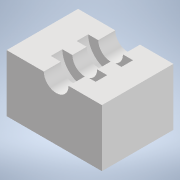
# Autodesk Inventor part: new_box_bottom
Saved by Autodesk Inventor 2021 (Build 250183000, 183)
## iProperties
Created: 2021-02-09
Part Number: new_box_bottom
Material: Generic
Document SubType Name: Modeling
Designer: user
Density: 1 g/cm^3
Appearance: Default
Author: user
Autodesk Inventor part; units mm, degrees
ref_plane "YZ Plane" through (0, 0, 0) normal (1, 0, 0) x (0, 1, 0)
ref_plane "XZ Plane" through (0, 0, 0) normal (0, 1, 0) x (-1, 0, 0)
ref_plane "XY Plane" through (0, 0, 0) normal (0, 0, 1) x (1, 0, 0)
sketch "Sketch1" plane through (0, 0, 0) normal (0, 1, 0) x (-1, 0, 0)
  line L0 (52, 58.6471) -> (-48, 58.6471)
  line L1 (-48, 58.6471) -> (-48, -16.3529)
  line L2 (-48, -16.3529) -> (52, -16.3529)
  line L3 (52, -16.3529) -> (52, 58.6471)
  point P0 (0, 0)
  dimension "d0" = 100
  dimension "d1" = 75
  constraints: 8 end point, 2 parallel, 1 horizontal, 1 perpendicular
  measures "d0" distance of L0.end L0.start
  measures "d1" distance of L1.end L0.end
extrude "Extrusion1" add sketch "Sketch1" along normal blind 60
sketch "Sketch2" plane through (0, 60, 0) normal (0, 1, 0) x (1, 0, 0)
  line L0 (-47, -53.6471) -> (43, -53.6471)
  line L1 (43, -53.6471) -> (43, 11.3529)
  line L2 (43, 11.3529) -> (-47, 11.3529)
  line L3 (-47, 11.3529) -> (-47, -53.6471)
  line L4 (-52, 16.3529) -> (-52, -58.6471) projected
  line L5 (-52, -58.6471) -> (48, -58.6471) projected
  line L6 (48, 16.3529) -> (-52, 16.3529) projected
  line L7 (48, -58.6471) -> (48, 16.3529) projected
  point P0 (0, 0)
  dimension "d4" = 5
  dimension "d5" = 5
  dimension "d6" = 5
  dimension "d7" = 5
  constraints: 8 end point, 2 parallel, 1 horizontal, 1 perpendicular
  measures "d4" distance from line of L4 L0.start
  measures "d5" distance between parallel lines of L5 L0
  measures "d6" distance between parallel lines of L6 L2
  measures "d7" distance between parallel lines of L7 L1
extrude "Extrusion2" cut sketch "Sketch2" against normal blind 59 contours L3 L2 L1 L0
sketch "Sketch3" plane through (48, 0, -16.3529) normal (0, 0, -1) x (-1, 0, 0)
  circle A0 centre (48, 60) radius 13
  point P0 (48, 0)
  dimension "d10" = 26
  dimension "d11" = 60
  constraints: 1 centre point
  measures "d10" diameter of A0
  measures "d11" distance of point (48, 0) A0.centre
sketch "Sketch13" plane through (0, 1, 0) normal (0, 1, 0) x (1, 0, 0)
  line L0 (-47, -53.6471) -> (-47, 11.3529) projected
  line L1 (43, 11.3529) -> (43, -53.6471) projected
  line L2 (-47, 11.3529) -> (43, 11.3529)
  line L3 (43, 11.3529) -> (43, -13.6471)
  line L4 (43, -13.6471) -> (-47, -13.6471)
  line L5 (-47, -13.6471) -> (-47, 11.3529)
  point P0 (0, 0)
  dimension "d44" = 25
  constraints: 8 end point, 2 parallel, 1 horizontal, 1 perpendicular, 1 point on line
  measures "d44" distance between parallel lines of L2 L4
extrude "Extrusion14" add sketch "Sketch13" along normal blind 59
sketch "Sketch14" plane through (-47, 1, 13.6471) normal (0, 0, 1) x (1, 0, 0)
  line L0 (0, 59) -> (90, 59) projected
  circle A0 centre (47, 59) radius 23.505
  point P0 (47, -1)
  dimension "d47" = 47.01
  constraints: 1 centre point, 1 point on line
  measures "d47" diameter of A0
extrude "Extrusion15" cut sketch "Sketch14" against normal blind 12.1
sketch "Sketch15" plane through (0, 1, 0) normal (0, 1, 0) x (1, 0, 0)
  line L0 (-47, -53.6471) -> (-47, -13.6471) projected
  line L1 (43, -13.6471) -> (43, -53.6471) projected
  line L2 (-47, -53.6471) -> (43, -53.6471)
  line L3 (43, -53.6471) -> (43, -28.6471)
  line L4 (43, -28.6471) -> (-47, -28.6471)
  line L5 (-47, -28.6471) -> (-47, -53.6471)
  point P0 (0, 0)
  point P1 (-47, -28.6471)
  dimension "d50" = 25
  constraints: 8 end point, 2 parallel, 1 horizontal, 1 perpendicular, 1 point on line
  measures "d50" distance between parallel lines of L4 L2
extrude "Extrusion16" add sketch "Sketch15" along normal blind 59
sketch "Sketch16" plane through (43, 1, 28.6471) normal (0, 0, -1) x (-1, 0, 0)
  line L0 (0, 59) -> (90, 59) projected
  circle A0 centre (43, 59) radius 23.505
  point P0 (43, -1)
  dimension "d53" = 47.01
  constraints: 1 centre point, 1 point on line
  measures "d53" diameter of A0
extrude "Extrusion17" cut sketch "Sketch16" against normal blind 12.1
sketch "Sketch17" plane through (0, 1, 0) normal (0, 1, 0) x (1, 0, 0)
  line L0 (23.505, -13.6471) -> (43, -13.6471) projected
  line L1 (-47, -28.6471) -> (43, -28.6471)
  line L2 (43, -28.6471) -> (43, -13.6471)
  line L3 (43, -13.6471) -> (-47, -13.6471)
  line L4 (-47, -13.6471) -> (-47, -28.6471)
  point P0 (0, 0)
  constraints: 8 end point, 2 parallel, 1 horizontal, 1 perpendicular
extrude "Extrusion18" add sketch "Sketch17" along normal blind 59
extrude "Extrusion19" cut sketch "Sketch3" against normal blind 75
equation "\"d6\" = d5"
equation "\"d7\" = d4"
body "Solid2"
